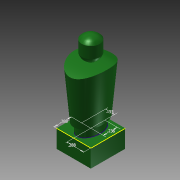
# Autodesk Inventor part: Automoblox MaleDE
Saved by Autodesk Inventor 2015 (Build 190159000, 159)
## iProperties
Created: 2018-01-03
Part Number: Automoblox MaleDE
Material: ABS Plastic
Document SubType Name: Modeling
Designer: Administrator
Density: 1.06 g/cm^3
Appearance: Smooth - Dark Forest Green
Mass: 5.87999 g
Surface Area: 23.3323 cm^2
Volume: 5.54716 cm^3
Author: Administrator
Autodesk Inventor part; units mm, degrees
ref_plane "YZ Plane" through (0, 0, 0) normal (1, 0, 0) x (0, 1, 0)
ref_plane "XZ Plane" through (0, 0, 0) normal (0, 1, 0) x (-1, 0, 0)
ref_plane "XY Plane" through (0, 0, 0) normal (0, 0, 1) x (1, 0, 0)
sketch "Sketch1" plane through (0, 0, 0) normal (0, 1, 0) x (-1, 0, 0)
  line L0 (0, 0) -> (14.605, 0)
  line L1 (14.605, 0) -> (14.605, -14.605)
  line L2 (14.605, -14.605) -> (0, -14.605)
  line L3 (0, -14.605) -> (0, 0)
  dimension "d0" = 14.605
  dimension "d1" = 14.605
  constraints: 8 end point, 2 parallel, 1 horizontal, 1 perpendicular
  measures "d0" distance of L0.start L0.end
  measures "d1" distance of L2.end L0.start
extrude "Extrusion1" add sketch "Sketch1" along normal blind 7.62
sketch "Sketch2" plane through (0, 7.62, 0) normal (0, 1, 0) x (1, 0, 0)
  line L0 (-14.605, 0) -> (0, 0) projected
  line L1 (0, 0) -> (0, 14.605) projected
  ellipse E0 centre (-7.3025, 7.3025) end of major axis (-7.3025, 13.2969) minor radius 3.937
  dimension "d6" = 5.9944
  dimension "d7" = 3.937
  dimension "d4" = 7.3025
  dimension "d5" = 7.3025
  constraints: 1 coincident, 2 other
  measures "d4" distance from line of L0 point (-7.303, 7.302)
  measures "d5" distance from line of L1 point (-7.303, 7.302)
extrude "Extrusion2" add sketch "Sketch2" along normal blind 3.937
sketch "Sketch3" plane through (0, 11.557, 0) normal (0, 1, 0) x (1, 0, 0)
  line L0 (-14.605, 0) -> (0, 0) projected
  line L1 (0, 0) -> (0, 14.605) projected
  ellipse E0 centre (-7.3025, 7.3025) end of major axis (-7.3025, 14.5669) minor radius 5.207
  dimension "d12" = 7.2644
  dimension "d13" = 5.207
  dimension "d10" = 7.3025
  dimension "d11" = 7.3025
  constraints: 1 coincident, 2 other
  measures "d10" distance from line of L0 point (-7.303, 7.302)
  measures "d11" distance from line of L1 point (-7.303, 7.302)
extrude "Extrusion3" add sketch "Sketch3" along normal blind 21.336 draft 5
ref_plane "Work Plane2" through (-7.3025, 0, 0) normal (1, 0, 0) x (0, 0, -1)
sketch "Sketch4" plane through (-7.3025, 0, 0) normal (1, 0, 0) x (0, 0, -1)
  line L0 (0, 0) -> (14.605, 0)
  line L1 (0, 0) -> (14.605, 0) projected
  line L2 (14.605, 0) -> (22.5425, 26.67)
  line L3 (13.2969, 11.557) -> (1.3081, 11.557) projected
  line L4 (0, 0) -> (-7.9375, 26.67)
  line L5 (-7.9375, 26.67) -> (22.5425, 26.67)
  arc A0 (22.5425, 26.67) -> (-7.9375, 26.67) centre (7.3025, 10.7378) ccw
  point P0 (7.3025, 0)
  dimension "d16" = 30.48
  dimension "d17" = 15.24
  dimension "d18" = 26.67
  constraints: 8 end point, 2 point on circle, 1 centre point, 1 collinear, 1 horizontal, 1 midpoint
  measures "d16" distance of L4.end L2.end
  measures "d17" horizontal distance of point (7.303, 0) L4.end
  measures "d18" distance from line of point (7.303, 0) L5
extrude "Extrusion4" cut sketch "Sketch4" along normal mid plane 25.4 keep common part
sketch "Sketch5" plane through (-7.3025, 0, 0) normal (1, 0, 0) x (0, 0, -1)
  line L0 (0.0381, 11.557) -> (14.5669, 11.557) projected
  line L1 (0, 7.62) -> (14.605, 7.62) projected
  line L2 (14.605, 0) -> (0, 0) projected
  line L3 (14.605, 0) -> (0, 0) projected
  line L4 (14.605, 0) -> (14.605, 7.62) projected
  line L5 (0, 7.62) -> (14.605, 7.62) projected
  line L6 (0, 0) -> (0, 7.62) projected
  line L7 (13.2969, 11.557) -> (1.3081, 11.557) projected
  line L8 (1.3081, 7.62) -> (13.2969, 7.62) projected
  arc A0 (11.1125, 40.5965) -> (7.3025, 42.3965) centre (7.3135, 37.4874) ccw
  line L9 (7.3025, 42.3965) -> (7.3025, 32.7424)
  line L10 (11.1125, 40.5965) -> (11.1125, 35.765)
  arc A1 (7.3025, 32.7424) -> (11.1125, 35.765) centre (7.3545, 36.5895) ccw
  constraints: 4 end point, 4 point on circle, 2 centre point, 2 vertical
revolve "Revolution1" add sketch "Sketch5" angle 360 about axis through (-7.3025, 42.3965, -7.3025) along (0, -1, 0) contours L10 A1 L9 A0
body "Solid1"
